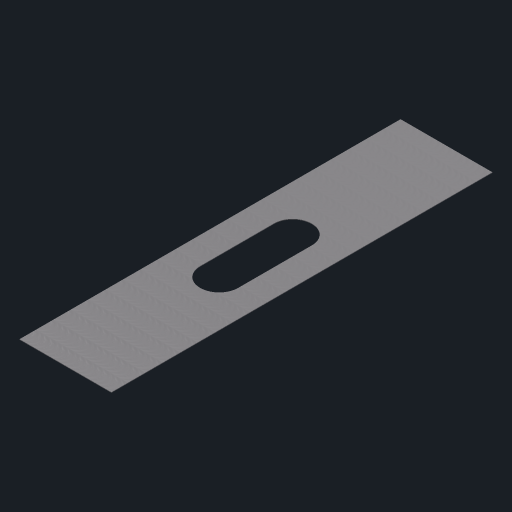
# Autodesk Inventor part: CHAPA_1
Saved by Autodesk Inventor 2024.3 (Build 283343000, 343)
## iProperties
Created: 2024-06-14
Part Number: CHAPA_1
Material: Steel, Mild, Welded
Document SubType Name: Sheet Metal
Designer: Niler
Density: 7.85 g/cm^3
Sheet Metal Rule: Default_mm
Appearance: Weld - Steel Mild
Flat Pattern Width: 23.7 cm
Flat Pattern Length: 98.3 cm
Flat Pattern Area: 2329.71 cm^2
Sheet Metal Width: 237.000 mm
Sheet Metal Length: 983.000 mm
Sheet Metal Area: 232971.000 mm^2
Author: Niler
Autodesk Inventor part; units mm, degrees
ref_plane "YZ Plane" through (0, 0, 0) normal (1, 0, 0) x (0, 1, 0)
ref_plane "XZ Plane" through (0, 0, 0) normal (0, 1, 0) x (-1, 0, 0)
ref_plane "XY Plane" through (0, 0, 0) normal (0, 0, 1) x (1, 0, 0)
sketch "Sketch1" plane through (0, 0, 0) normal (0, 1, 0) x (-1, 0, 0)
  line L0 (-118.5, 491.5) -> (118.5, 491.5)
  line L1 (118.5, 491.5) -> (118.5, -491.5)
  line L2 (118.5, -491.5) -> (-118.5, -491.5)
  line L3 (-118.5, -491.5) -> (-118.5, 491.5)
  line L4 (-118.5, 491.5) -> (118.5, -491.5) construction
  line L5 (118.5, 491.5) -> (-118.5, -491.5) construction
  point P0 (0, 0)
  dimension "d0" = 983
  dimension "d1" = 237
extrude "Plate1" add sketch "Sketch1" along normal blind 1.5
sketch "Sketch2" plane through (0, 1.5, 0) normal (0, 1, 0) x (1, 0, 0)
  line L0 (0, -95) -> (0, 95) construction
  line L1 (49, -95) -> (49, 95)
  line L2 (-49, 95) -> (-49, -95)
  arc A0 (-49, -95) -> (49, -95) centre (0, -95) ccw
  arc A1 (49, 95) -> (-49, 95) centre (0, 95) ccw
  point P0 (0, 0)
  point P1 (0, 144)
  point P2 (0, -144)
  dimension "d17" = 98
  dimension "d19" = 190
  constraints: 8 end point, 6 point on circle, 4 tangent, 2 centre point, 1 midpoint, 1 parallel, 1 vertical
  measures "d17" distance between parallel lines of L1 L2
  measures "d19" distance of L0.start L0.end
extrude "Extrusion1" cut sketch "Sketch2" against normal through all
equation "\"d2\" = Thickness"
equation "\"BendRadius\" = Thickness"
equation "\"BendReliefWidth\" = Thickness"
equation "\"BendReliefDepth\" = 0.5 * Thickness"
equation "\"CornerReliefSize\" = 4 * Thickness"
equation "\"MinimumRemnant\" = 2 * Thickness"
equation "\"TransitionRadius\" = BendRadius"
equation "\"JacobiRadiusSize\" = BendRadius"
equation "\"GapSize\" = Thickness"
equation "\"Thickness\" = 1.5"
body "Solid1"
